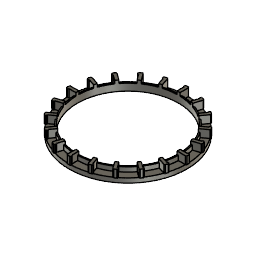
FanRing (Autodesk Fusion 360 design; units mm, degrees)
Autodesk Fusion 360 part; units mm, degrees
sketch "Sketch1" plane through (0, 0, 0) normal (0, 0, 1) x (1, 0, 0)
  circle A0 centre (0, 0) radius 36.8
  circle A1 centre (0, 0) radius 38.5
  circle A2 centre (0, 0) radius 33
  dimension "d1" = 73.6
  dimension "d2" = 77
  dimension "d3" = 66
  constraint coincident A0.centre A1.centre
  constraint concentric A0 A1
  measures "d1" diameter of A0
  measures "d2" diameter of A1
  measures "d3" diameter of A2
extrude "Extrude1" add sketch "Sketch1" against normal blind 1.5 contours A1
extrude "Extrude2" add sketch "Sketch1" along normal blind 1.5 contours A0 | A1
sketch "Sketch2" plane through (0, 0, 1.5) normal (0, 0, 1) x (-1, 0, 0)
  circle A0 centre (0, 0) radius 33
  circle A1 centre (0, 0) radius 38.5
  circle A2 centre (0, 0) radius 33.85
  dimension "d8" = 67.7
  constraint concentric A0 A2
  measures "d8" diameter of A2
extrude "Extrude3" add sketch "Sketch2" along normal blind 3 contours A2
sketch "Sketch3" plane through (0, 0, 1.5) normal (0, 0, 1) x (-1, 0, 0)
  circle A0 centre (0, 0) radius 33.85
  circle A1 centre (0, 0) radius 38.5
  line L0 (-1, 32) -> (1, 32)
  line L1 (1, 32) -> (-1, 32)
  line L2 (-1, 32) -> (-1, 39)
  line L3 (-1, 39) -> (0.5, 39)
  line L4 (1, 38.5) -> (1, 32)
  line L5 (-1.5, 38) -> (-1.5, 38.5)
  line L6 (-1, 39) -> (-1, 37.5)
  arc A2 (1, 38.5) -> (0.5, 39) centre (0.5, 38.5) ccw
  arc A3 (-1, 39) -> (-1.5, 38.5) centre (-1, 38.5) ccw
  arc A4 (-1.5, 38) -> (-1, 37.5) centre (-1, 38) ccw
  point P0 (0, 32)
  point P1 (-1, 38.487)
  dimension "d11" = 0.5
  constraint midpoint L0 P0
  constraint horizontal L0
  constraint horizontal L1
  constraint vertical L2
  constraint horizontal L3
  constraint vertical L4
  constraint coincident A1 P1
  constraint coincident L2 P1
  constraint vertical L5
  constraint vertical L6
  constraint coincident L2 L6.end
  constraint tangent L4 A2
  constraint tangent L3 A2
  constraint tangent L5 A3
  constraint equal A2 A3
  constraint coincident L2.end L3.start
  constraint tangent L5 A4
  constraint equal A2 A4
  constraint coincident L6.end A4.end
  measures "d11" radius of A2
extrude "Extrude4" add sketch "Sketch3" along normal blind 5 contours A0 A1 L2 L4 L6 | A1 L2 L3 L4 L6 A2 | A1 L2 L5 L6 A4 | A1 L2 L5 L6 A3
pattern_circular "C-Pattern1" count 20 over 360 about axis through (0, 0, 1.75) along (0, 0, 1) of "Extrude4"
sketch "Sketch4" plane through (0, 0, 4.5) normal (0, 0, 1) x (-1, 0, 0)
  circle A0 centre (0, 0) radius 33
  arc A1 (-1, 33.8352) -> (-9.5046, 32.4882) centre (0, 0) ccw
  arc A2 (-9.5046, 32.4882) -> (-11.4067, 31.8702) centre (0, 0) ccw
  arc A3 (-11.4067, 31.8702) -> (-19.0788, 27.9611) centre (0, 0) ccw
  arc A4 (-19.0788, 27.9611) -> (-20.6969, 26.7855) centre (0, 0) ccw
  arc A5 (-20.6969, 26.7855) -> (-26.7855, 20.6969) centre (0, 0) ccw
  arc A6 (-26.7855, 20.6969) -> (-27.9611, 19.0788) centre (0, 0) ccw
  arc A7 (-27.9611, 19.0788) -> (-31.8702, 11.4067) centre (0, 0) ccw
  arc A8 (-31.8702, 11.4067) -> (-32.4882, 9.5046) centre (0, 0) ccw
  arc A9 (-32.4882, 9.5046) -> (-33.8352, 1) centre (0, 0) ccw
  arc A10 (-33.8352, 1) -> (-33.8352, -1) centre (0, 0) ccw
  arc A11 (-33.8352, -1) -> (-32.4882, -9.5046) centre (0, 0) ccw
  arc A12 (-32.4882, -9.5046) -> (-31.8702, -11.4067) centre (0, 0) ccw
  arc A13 (-31.8702, -11.4067) -> (-27.9611, -19.0788) centre (0, 0) ccw
  arc A14 (-27.9611, -19.0788) -> (-26.7855, -20.6969) centre (0, 0) ccw
  arc A15 (-26.7855, -20.6969) -> (-20.6969, -26.7855) centre (0, 0) ccw
  arc A16 (-20.6969, -26.7855) -> (-19.0788, -27.9611) centre (0, 0) ccw
  arc A17 (-19.0788, -27.9611) -> (-11.4067, -31.8702) centre (0, 0) ccw
  arc A18 (-11.4067, -31.8702) -> (-9.5046, -32.4882) centre (0, 0) ccw
  arc A19 (-9.5046, -32.4882) -> (-1, -33.8352) centre (0, 0) ccw
  arc A20 (-1, -33.8352) -> (1, -33.8352) centre (0, 0) ccw
  arc A21 (1, -33.8352) -> (9.5046, -32.4882) centre (0, 0) ccw
  arc A22 (9.5046, -32.4882) -> (11.4067, -31.8702) centre (0, 0) ccw
  arc A23 (11.4067, -31.8702) -> (19.0788, -27.9611) centre (0, 0) ccw
  arc A24 (19.0788, -27.9611) -> (20.6969, -26.7855) centre (0, 0) ccw
  arc A25 (20.6969, -26.7855) -> (26.7855, -20.6969) centre (0, 0) ccw
  arc A26 (26.7855, -20.6969) -> (27.9611, -19.0788) centre (0, 0) ccw
  arc A27 (27.9611, -19.0788) -> (31.8702, -11.4067) centre (0, 0) ccw
  arc A28 (31.8702, -11.4067) -> (32.4882, -9.5046) centre (0, 0) ccw
  arc A29 (32.4882, -9.5046) -> (33.8352, -1) centre (0, 0) ccw
  arc A30 (33.8352, -1) -> (33.8352, 1) centre (0, 0) ccw
  arc A31 (33.8352, 1) -> (32.4882, 9.5046) centre (0, 0) ccw
  arc A32 (32.4882, 9.5046) -> (31.8702, 11.4067) centre (0, 0) ccw
  arc A33 (31.8702, 11.4067) -> (27.9611, 19.0788) centre (0, 0) ccw
  arc A34 (27.9611, 19.0788) -> (26.7855, 20.6969) centre (0, 0) ccw
  arc A35 (26.7855, 20.6969) -> (20.6969, 26.7855) centre (0, 0) ccw
  arc A36 (20.6969, 26.7855) -> (19.0788, 27.9611) centre (0, 0) ccw
  arc A37 (19.0788, 27.9611) -> (11.4067, 31.8702) centre (0, 0) ccw
  arc A38 (11.4067, 31.8702) -> (9.5046, 32.4882) centre (0, 0) ccw
  arc A39 (9.5046, 32.4882) -> (1, 33.8352) centre (0, 0) ccw
  arc A40 (1, 33.8352) -> (-1, 33.8352) centre (0, 0) ccw
  line L0 (1, 32.5) -> (-1, 32.5)
  line L1 (-1, 32.5) -> (-1, 34)
  line L2 (-1, 34) -> (1, 34)
  line L3 (1, 34) -> (1, 32.5)
  constraint horizontal L0
  constraint vertical L1
  constraint horizontal L2
  constraint vertical L3
extrude "Extrude5" add sketch "Sketch4" along normal blind 2 contours A0 A40 L1 L3
pattern_circular "C-Pattern2" count 20 over 360 about axis through (0, 0, 1.75) along (0, 0, 1) of "Extrude5"
